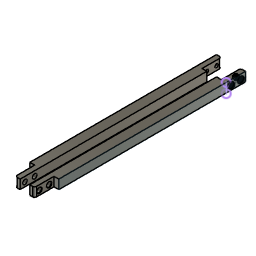
Base_Extension (Autodesk Fusion 360 design; units mm, degrees)
Autodesk Fusion 360 part; units mm, degrees
note: some values were not read from the file. Set by a fixed rule: which sketch regions a step uses.
sketch "Sketch1" plane through (0, 0, 0) normal (0, 0, 1) x (1, 0, 0)
  line L0 (0, 0) -> (5, 0) construction
  line L1 (5, 0) -> (5, -193)
  line L2 (5, -193) -> (10, -193)
  line L3 (10, -193) -> (10, -173)
  line L4 (10, -173) -> (15, -173)
  line L5 (15, -173) -> (15, 20)
  line L6 (10, 0) -> (5, 0)
  line L7 (10, 0) -> (10, 20)
  line L8 (10, 20) -> (15, 20)
  dimension "d1" = 5
  dimension "d3" = 5
  dimension "d5" = 5
  dimension "d8" = 20
  dimension "d16" = 20
  dimension "d17" = 5
  dimension "d36" = 173
  constraint coincident L0.start origin
  constraint horizontal L0
  constraint perpendicular L0 L1
  constraint perpendicular L1 L2
  constraint perpendicular L2 L3
  constraint perpendicular L3 L4
  constraint perpendicular L2 L5
  constraint perpendicular L1 L6
  constraint perpendicular L6 L7
  constraint perpendicular L7 L8
  constraint coincident L5.end L8
  constraint coincident L5.end L8.end
  measures "d1" distance of L0.start L0.end
  measures "d3" distance of L1.end L2.end
  measures "d5" distance of L3.end L4.end
  measures "d8" distance of L2.end L3.end
  measures "d16" distance of L6.start L7.end
  measures "d17" distance of L7.end L5.end
  measures "d36" distance of L4 L6
extrude "Extrude1" add sketch "Sketch1" along normal blind 10 makes body 1
sketch "Sketch5" plane through (10, 0, 0) normal (1, 0, 0) x (0, 1, 0)
  line L0 (-193, 0) -> (-173, 0)
  line L1 (-173, 0) -> (-173, 10)
  line L2 (-173, 10) -> (-193, 10)
  line L3 (-193, 10) -> (-193, 0)
  line L4 (-173, 5) -> (-193, 5) construction
  line L5 (-183, 5) -> (-183, 10) construction
  circle A0 centre (-178, 5) radius 2.35
  circle A1 centre (-188, 5) radius 2.35
  dimension "d27" = 4.7
  dimension "d29" = 5
  constraint midpoint L1 L4.start
  constraint midpoint L3 L4.end
  constraint midpoint L4 L5.start
  constraint midpoint L2 L5.end
  constraint coincident L4 A0.centre
  constraint symmetric L5 A0 A1
  measures "d27" diameter of A0
  measures "d29" distance of L1 A0.centre
extrude "Extrude6" cut sketch "Sketch5" against normal up to surface (5 mm away) contours A0 | A1 bodies 1
sketch "Sketch4" plane through (15, 0, 0) normal (1, 0, 0) x (0, 1, 0)
  line L0 (-173, 0) -> (20, 0)
  line L1 (20, 0) -> (20, 10)
  line L2 (20, 10) -> (-173, 10)
  line L3 (-173, 10) -> (-173, 0)
  line L4 (0, 0) -> (0, 10)
  line L5 (0, 5) -> (20, 5) construction
  line L6 (10, 5) -> (10, 10) construction
  circle A0 centre (5, 5) radius 1.75
  circle A1 centre (5, 5) radius 3
  circle A2 centre (15, 5) radius 3
  circle A3 centre (15, 5) radius 1.75
  dimension "d18" = 3.5
  dimension "d19" = 6
  dimension "d20" = 5
  constraint midpoint L4 L5.start
  constraint midpoint L1 L5.end
  constraint midpoint L5 L6.start
  constraint coincident L2 L6.end
  constraint perpendicular L2 L6
  constraint coincident L5 A0.centre
  constraint concentric A0 A1
  constraint symmetric L6 A0 A3
  constraint symmetric L6 A1 A2
  measures "d18" diameter of A0
  measures "d19" diameter of A1
  measures "d20" distance of L4 A0.centre
extrude "Extrude4" cut sketch "Sketch4" against normal up to surface (5 mm away) contours A0 | A3 bodies 1
extrude "Extrude5" cut sketch "Sketch4" against normal blind 3 contours A1 | A2 bodies 1
chamfer "Chamfer1" distance 0.4 angle 45 2 edges at (10, -190.191, 5.8498) (10, -180.191, 5.8498) on bodies 1
fillet "Fillet1" radius 2 2 edges at (10, -193, 5) (10, 20, 5) on bodies 1
chamfer "Chamfer2" distance 0.6 angle 45 1 faces at (6.6667, -122, 0) on bodies 1
mirror "Mirror1" about plane through (0, 0, 0) normal (1, 0, 0) of bodies 1 makes body 2
